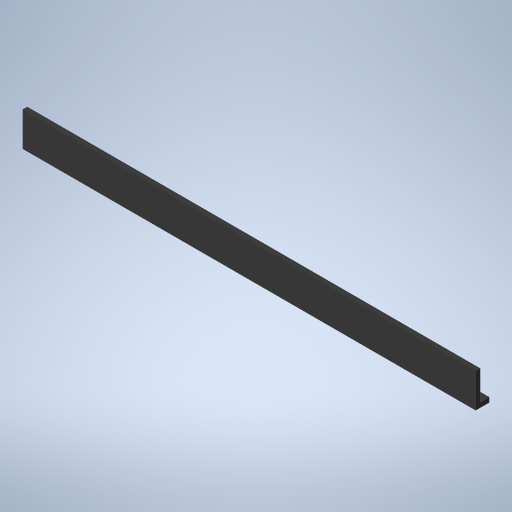
# Autodesk Inventor part: GuiderailRS3
Saved by Autodesk Inventor 2024.3 (Build 283343000, 343)
## iProperties
Created: 2025-08-09
Part Number: GuiderailRS3
Material: Generic
Document SubType Name: Modeling
Designer: ajclo
Density: 1 g/cm^3
Appearance: Default
Author: ajclo
Autodesk Inventor part; units mm, degrees
ref_plane "YZ Plane" through (0, 0, 0) normal (1, 0, 0) x (0, 1, 0)
ref_plane "XZ Plane" through (0, 0, 0) normal (0, 1, 0) x (-1, 0, 0)
ref_plane "XY Plane" through (0, 0, 0) normal (0, 0, 1) x (1, 0, 0)
sketch "Sketch1" plane through (0, 0, 0) normal (1, 0, 0) x (0, 1, 0)
  line L0 (0, 0) -> (15, 0)
  line L1 (15, 0) -> (15, -2)
  line L2 (15, -2) -> (0, -2)
  line L3 (0, -2) -> (0, 0)
  line L4 (0, 0) -> (2, 0)
  line L5 (2, 0) -> (2, -6)
  line L6 (2, -6) -> (0, -6)
  line L7 (0, -6) -> (0, 0)
  point P0 (0, -1)
  point P1 (1, 0)
  point P2 (1, -6)
  point P3 (2, -2)
  point P4 (0, -2)
  dimension "d0" = 15
  dimension "d1" = 2
  dimension "d2" = 2
  dimension "d3" = 6
  constraints: 16 end point, 4 parallel, 3 midpoint, 2 horizontal, 2 perpendicular
  measures "d0" distance of L0.start L0.end
  measures "d1" distance between parallel lines of L2 L0
  measures "d2" distance from line of point (0, -1) L5
  measures "d3" distance of point (1, 0) point (1, -6)
extrude "Extrusion1" add sketch "Sketch1" along normal blind 200
equation "\"d2\" = d1"
body "Solid1"
